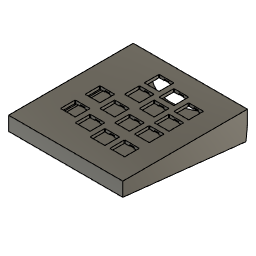
fdmyouA (Autodesk Fusion 360 design; units mm, degrees)
Autodesk Fusion 360 part; units mm, degrees
(part 1 of 2)
sketch "スケッチ1" plane through (0, 0, 0) normal (0, 0, 1) x (1, 0, 0)
  arc A0 (50.4, -11.9) -> (49.9, -12.4) centre (50.4, -12.4) ccw
  arc A1 (64.1, -12.4) -> (63.6, -11.9) centre (63.6, -12.4) ccw
  line L0 (31.4, -7.15) -> (44.6, -7.15)
  line L1 (45.1, -7.65) -> (45.1, -20.85)
  line L2 (50.4, -11.9) -> (63.6, -11.9)
  line L3 (31.4, -21.35) -> (44.6, -21.35)
  line L4 (64.1, -12.4) -> (64.1, -25.6)
  arc A2 (44.6, -21.35) -> (45.1, -20.85) centre (44.6, -20.85) ccw
  arc A3 (31.4, -7.15) -> (30.9, -7.65) centre (31.4, -7.65) ccw
  arc A4 (45.1, -7.65) -> (44.6, -7.15) centre (44.6, -7.65) ccw
  line L5 (49.9, -12.4) -> (49.9, -25.6)
  arc A5 (30.9, -20.85) -> (31.4, -21.35) centre (31.4, -20.85) ccw
  arc A6 (82.6, -30.85) -> (83.1, -30.35) centre (82.6, -30.35) ccw
  line L6 (50.4, -26.1) -> (63.6, -26.1)
  line L7 (83.1, -17.15) -> (83.1, -30.35)
  line L8 (30.9, -26.65) -> (30.9, -39.85)
  line L9 (45.1, -26.65) -> (45.1, -39.85)
  line L10 (50.4, -30.9) -> (63.6, -30.9)
  line L11 (30.9, -7.65) -> (30.9, -20.85)
  arc A7 (64.1, -31.4) -> (63.6, -30.9) centre (63.6, -31.4) ccw
  line L12 (69.4, -35.65) -> (82.6, -35.65)
  arc A8 (45.1, -26.65) -> (44.6, -26.15) centre (44.6, -26.65) ccw
  arc A9 (68.9, -30.35) -> (69.4, -30.85) centre (69.4, -30.35) ccw
  line L13 (68.9, -17.15) -> (68.9, -30.35)
  arc A10 (63.6, -26.1) -> (64.1, -25.6) centre (63.6, -25.6) ccw
  line L14 (49.9, -31.4) -> (49.9, -44.6)
  arc A11 (83.1, -17.15) -> (82.6, -16.65) centre (82.6, -17.15) ccw
  arc A12 (30.9, -39.85) -> (31.4, -40.35) centre (31.4, -39.85) ccw
  line L15 (69.4, -16.65) -> (82.6, -16.65)
  line L16 (69.4, -49.85) -> (82.6, -49.85)
  line L17 (69.4, -30.85) -> (82.6, -30.85)
  line L18 (68.9, -36.15) -> (68.9, -49.35)
  arc A13 (69.4, -35.65) -> (68.9, -36.15) centre (69.4, -36.15) ccw
  line L19 (64.1, -31.4) -> (64.1, -44.6)
  line L20 (83.1, -36.15) -> (83.1, -49.35)
  arc A14 (83.1, -36.15) -> (82.6, -35.65) centre (82.6, -36.15) ccw
  arc A15 (68.9, -49.35) -> (69.4, -49.85) centre (69.4, -49.35) ccw
  arc A16 (50.4, -30.9) -> (49.9, -31.4) centre (50.4, -31.4) ccw
  arc A17 (63.6, -45.1) -> (64.1, -44.6) centre (63.6, -44.6) ccw
  arc A18 (82.6, -49.85) -> (83.1, -49.35) centre (82.6, -49.35) ccw
  line L21 (12.4, -45.15) -> (25.6, -45.15)
  arc A19 (69.4, -16.65) -> (68.9, -17.15) centre (69.4, -17.15) ccw
  arc A20 (44.6, -40.35) -> (45.1, -39.85) centre (44.6, -39.85) ccw
  line L22 (31.4, -26.15) -> (44.6, -26.15)
  arc A21 (31.4, -26.15) -> (30.9, -26.65) centre (31.4, -26.65) ccw
  arc A22 (49.9, -25.6) -> (50.4, -26.1) centre (50.4, -25.6) ccw
  arc A23 (49.9, -44.6) -> (50.4, -45.1) centre (50.4, -44.6) ccw
  line L23 (31.4, -40.35) -> (44.6, -40.35)
  line L24 (50.4, -92.6) -> (63.6, -92.6)
  line L25 (49.9, -55.15) -> (49.9, -68.35)
  line L26 (69.4, -54.65) -> (82.6, -54.65)
  arc A24 (82.6, -92.6) -> (83.1, -92.1) centre (82.6, -92.1) ccw
  line L27 (83.1, -55.15) -> (83.1, -68.35)
  arc A25 (26.1, -69.4) -> (25.6, -68.9) centre (25.6, -69.4) ccw
  arc A26 (44.6, -87.85) -> (45.1, -87.35) centre (44.6, -87.35) ccw
  line L28 (64.1, -55.15) -> (64.1, -68.35)
  arc A27 (31.4, -49.9) -> (30.9, -50.4) centre (31.4, -50.4) ccw
  arc A28 (11.9, -58.85) -> (12.4, -59.35) centre (12.4, -58.85) ccw
  line L29 (31.4, -64.1) -> (44.6, -64.1)
  line L30 (69.4, -68.85) -> (82.6, -68.85)
  arc A29 (30.9, -63.6) -> (31.4, -64.1) centre (31.4, -63.6) ccw
  line L31 (11.9, -45.65) -> (11.9, -58.85)
  line L32 (12.4, -68.9) -> (25.6, -68.9)
  arc A30 (12.4, -45.15) -> (11.9, -45.65) centre (12.4, -45.65) ccw
  line L33 (31.4, -49.9) -> (44.6, -49.9)
  line L34 (12.4, -83.1) -> (25.6, -83.1)
  arc A31 (26.1, -45.65) -> (25.6, -45.15) centre (25.6, -45.65) ccw
  line L35 (68.9, -55.15) -> (68.9, -68.35)
  arc A32 (11.9, -82.6) -> (12.4, -83.1) centre (12.4, -82.6) ccw
  arc A33 (45.1, -50.4) -> (44.6, -49.9) centre (44.6, -50.4) ccw
  arc A34 (44.6, -64.1) -> (45.1, -63.6) centre (44.6, -63.6) ccw
  line L36 (12.4, -59.35) -> (25.6, -59.35)
  arc A35 (82.6, -68.85) -> (83.1, -68.35) centre (82.6, -68.35) ccw
  arc A36 (68.9, -68.35) -> (69.4, -68.85) centre (69.4, -68.35) ccw
  arc A37 (49.9, -68.35) -> (50.4, -68.85) centre (50.4, -68.35) ccw
  line L37 (50.4, -54.65) -> (63.6, -54.65)
  arc A38 (63.6, -68.85) -> (64.1, -68.35) centre (63.6, -68.35) ccw
  line L38 (30.9, -74.15) -> (30.9, -87.35)
  arc A39 (31.4, -73.65) -> (30.9, -74.15) centre (31.4, -74.15) ccw
  arc A40 (64.1, -55.15) -> (63.6, -54.65) centre (63.6, -55.15) ccw
  line L39 (31.4, -87.85) -> (44.6, -87.85)
  arc A41 (50.4, -54.65) -> (49.9, -55.15) centre (50.4, -55.15) ccw
  line L40 (26.1, -45.65) -> (26.1, -58.85)
  line L41 (45.1, -74.15) -> (45.1, -87.35)
  line L42 (45.1, -50.4) -> (45.1, -63.6)
  line L43 (50.4, -68.85) -> (63.6, -68.85)
  line L44 (50.4, -78.4) -> (63.6, -78.4)
  arc A42 (69.4, -54.65) -> (68.9, -55.15) centre (69.4, -55.15) ccw
  arc A43 (45.1, -74.15) -> (44.6, -73.65) centre (44.6, -74.15) ccw
  line L45 (64.1, -78.9) -> (64.1, -92.1)
  arc A44 (50.4, -78.4) -> (49.9, -78.9) centre (50.4, -78.9) ccw
  arc A45 (12.4, -68.9) -> (11.9, -69.4) centre (12.4, -69.4) ccw
  arc A46 (25.6, -83.1) -> (26.1, -82.6) centre (25.6, -82.6) ccw
  arc A47 (25.6, -59.35) -> (26.1, -58.85) centre (25.6, -58.85) ccw
  line L46 (30.9, -50.4) -> (30.9, -63.6)
  arc A48 (83.1, -55.15) -> (82.6, -54.65) centre (82.6, -55.15) ccw
  line L47 (11.9, -69.4) -> (11.9, -82.6)
  line L48 (26.1, -69.4) -> (26.1, -82.6)
  line L49 (31.4, -73.65) -> (44.6, -73.65)
  line L50 (49.9, -78.9) -> (49.9, -92.1)
  arc A49 (64.1, -78.9) -> (63.6, -78.4) centre (63.6, -78.9) ccw
  arc A50 (30.9, -87.35) -> (31.4, -87.85) centre (31.4, -87.35) ccw
  line L51 (69.4, -92.6) -> (82.6, -92.6)
  arc A51 (63.6, -92.6) -> (64.1, -92.1) centre (63.6, -92.1) ccw
  line L52 (69.4, -78.4) -> (82.6, -78.4)
  line L53 (83.1, -78.9) -> (83.1, -92.1)
  arc A52 (69.4, -78.4) -> (68.9, -78.9) centre (69.4, -78.9) ccw
  arc A53 (49.9, -92.1) -> (50.4, -92.6) centre (50.4, -92.1) ccw
  arc A54 (68.9, -92.1) -> (69.4, -92.6) centre (69.4, -92.1) ccw
  line L54 (68.9, -78.9) -> (68.9, -92.1)
  arc A55 (83.1, -78.9) -> (82.6, -78.4) centre (82.6, -78.9) ccw
  line L55 (-2.5, -3.7) -> (97.5, -3.7)
  line L56 (-7.5, -3.7) -> (102.5, -3.7)
  line L57 (102.5, -3.7) -> (102.5, -113.7)
  line L58 (102.5, -113.7) -> (-7.5, -113.7)
  line L59 (-7.5, -113.7) -> (-7.5, -3.7)
  line L60 (47.5, -3.7) -> (47.5, -113.7)
  line L61 (47.5, -3.7) -> (42.3, -3.7)
  line L62 (47.5, -3.7) -> (-2.7, -3.7)
  line L63 (-2.7, -3.7) -> (97.7, -3.7)
  line L64 (97.7, -3.7) -> (97.7, -103.9)
  line L65 (97.7, -103.9) -> (-2.7, -103.9)
  line L66 (-2.7, -103.9) -> (-2.7, -3.7)
  line L67 (47.5, -3.7) -> (9.5, -3.7)
  line L68 (9.5, -3.7) -> (7.4071, -3.7)
  line L69 (-2.7, -3.7) -> (7.3, -3.7)
  line L70 (7.3, -3.7) -> (7.3, -103.9)
  line L71 (7.3, -103.9) -> (-2.7, -103.9)
  line L72 (-2.7, -103.9) -> (-2.7, 6.3)
  line L73 (-2.7, -103.9) -> (97.7, -103.9)
  line L74 (97.7, -103.9) -> (97.7, -93.9)
  line L75 (97.7, -93.9) -> (-2.7, -93.9)
  line L76 (-2.7, -93.9) -> (-2.7, -103.9)
  line L77 (97.7, -103.9) -> (87.7, -103.9)
  line L78 (87.7, -103.9) -> (87.7, -3.7)
  line L79 (87.7, -3.7) -> (97.7, -3.7)
  line L80 (97.7, -3.7) -> (97.7, -103.9)
  line L81 (40.1, -21.85) -> (35.9, -21.85)
  line L82 (35.9, -21.85) -> (35.9, -21.35)
  line L83 (40.1, -21.35) -> (40.1, -21.85)
  line L84 (40.1, -21.85) -> (38, -21.35) construction
  line L85 (35.9, -21.85) -> (38, -21.35) construction
  line L86 (38, -7.15) -> (40.1, -6.65) construction
  line L87 (38, -7.15) -> (35.9, -6.65) construction
  line L88 (40.1, -6.65) -> (40.1, -7.15)
  line L89 (35.9, -7.65) -> (35.9, -6.65)
  line L90 (35.9, -6.65) -> (40.1, -6.65)
  line L91 (35.9, -7.15) -> (35.9, -6.65)
  line L92 (38, -7.15) -> (40.1, -6.65) construction
  line L93 (35.9, -6.65) -> (40.1, -6.65)
  line L94 (38, -7.15) -> (35.9, -6.65) construction
  line L95 (40.1, -6.65) -> (40.1, -7.15)
  line L96 (54.9, -11.9) -> (54.9, -11.4)
  line L97 (57, -11.9) -> (59.1, -11.4) construction
  line L98 (54.9, -11.4) -> (59.1, -11.4)
  line L99 (57, -11.9) -> (54.9, -11.4) construction
  line L100 (59.1, -11.4) -> (59.1, -12.4)
  line L101 (54.9, -26.6) -> (54.9, -26.1)
  line L102 (54.9, -26.6) -> (57, -26.1) construction
  line L103 (59.1, -26.6) -> (54.9, -26.6)
  line L104 (59.1, -26.1) -> (59.1, -26.6)
  line L105 (73.9, -16.65) -> (73.9, -16.15)
  line L106 (76, -16.65) -> (78.1, -16.15) construction
  line L107 (73.9, -16.15) -> (78.1, -16.15)
  line L108 (76, -16.65) -> (73.9, -16.15) construction
  line L109 (78.1, -16.15) -> (78.1, -16.65)
  line L110 (73.9, -31.35) -> (73.9, -30.85)
  line L111 (73.9, -31.35) -> (76, -30.85) construction
  line L112 (78.1, -31.35) -> (73.9, -31.35)
  line L113 (78.1, -31.35) -> (76, -30.85) construction
  line L114 (78.1, -30.85) -> (78.1, -31.35)
  line L115 (35.9, -26.15) -> (35.9, -25.65)
  line L116 (38, -26.15) -> (40.1, -25.65) construction
  line L117 (35.9, -25.65) -> (40.1, -25.65)
  line L118 (38, -26.15) -> (35.9, -25.65) construction
  line L119 (40.1, -25.65) -> (40.1, -26.15)
  line L120 (35.9, -40.85) -> (35.9, -40.35)
  line L121 (40.1, -40.85) -> (35.9, -40.85)
  line L122 (40.1, -40.85) -> (38, -40.35) construction
  line L123 (40.1, -40.35) -> (40.1, -40.85)
  line L124 (54.9, -30.9) -> (54.9, -30.4)
  line L125 (57, -30.9) -> (59.1, -30.4) construction
  line L126 (54.9, -30.4) -> (59.1, -30.4)
  line L127 (57, -30.9) -> (54.9, -30.4) construction
  line L128 (59.1, -30.4) -> (59.1, -30.9)
  line L129 (54.9, -45.6) -> (54.9, -45.1)
  line L130 (54.9, -45.6) -> (57, -45.1) construction
  line L131 (59.1, -45.6) -> (54.9, -45.6)
  line L132 (59.1, -45.6) -> (57, -45.1) construction
  line L133 (59.1, -45.1) -> (59.1, -45.6)
  line L134 (73.9, -35.65) -> (73.9, -35.15)
  line L135 (76, -35.65) -> (78.1, -35.15) construction
  line L136 (73.9, -35.15) -> (78.1, -35.15)
  line L137 (76, -35.65) -> (73.9, -35.15) construction
  line L138 (78.1, -35.15) -> (78.1, -35.65)
  line L139 (73.9, -50.35) -> (73.9, -49.85)
  line L140 (73.9, -50.35) -> (76, -49.85) construction
  line L141 (78.1, -50.35) -> (73.9, -50.35)
  line L142 (78.1, -50.35) -> (76, -49.85) construction
  line L143 (78.1, -49.85) -> (78.1, -50.35)
  line L144 (16.9, -45.15) -> (16.9, -44.65)
  line L145 (16.9, -45.65) -> (21.1, -44.65) construction
  line L146 (16.9, -44.65) -> (21.1, -44.65)
  line L147 (19, -45.15) -> (16.9, -44.65) construction
  line L148 (21.1, -44.65) -> (21.1, -45.15)
  line L149 (16.9, -59.85) -> (16.9, -59.35)
  line L150 (16.9, -59.85) -> (19, -59.35) construction
  line L151 (21.1, -59.85) -> (16.9, -59.85)
  line L152 (21.1, -59.85) -> (19, -59.35) construction
  line L153 (21.1, -59.35) -> (21.1, -59.85)
  line L154 (35.9, -49.9) -> (35.9, -49.4)
  line L155 (38, -49.9) -> (40.1, -49.4) construction
  line L156 (35.9, -49.4) -> (40.1, -49.4)
  line L157 (38, -49.9) -> (35.9, -49.4) construction
  line L158 (40.1, -49.4) -> (40.1, -49.9)
  line L159 (35.9, -64.6) -> (35.9, -64.1)
  line L160 (35.9, -64.6) -> (38, -64.1) construction
  line L161 (40.1, -64.6) -> (35.9, -64.6)
  line L162 (40.1, -64.6) -> (38, -64.1) construction
  line L163 (40.1, -64.1) -> (40.1, -64.6)
  line L164 (54.9, -54.65) -> (54.9, -54.15)
  line L165 (57, -54.65) -> (59.1, -54.15) construction
  line L166 (54.9, -54.15) -> (59.1, -54.15)
  line L167 (57, -54.65) -> (54.9, -54.15) construction
  line L168 (59.1, -54.15) -> (59.1, -54.65)
  line L169 (54.9, -69.35) -> (54.9, -68.85)
  line L170 (54.9, -69.35) -> (57, -68.85) construction
  line L171 (59.1, -69.35) -> (54.9, -69.35)
  line L172 (59.1, -69.35) -> (57, -68.85) construction
  line L173 (59.1, -68.85) -> (59.1, -69.35)
  line L174 (73.9, -54.65) -> (73.9, -54.15)
  line L175 (73.9, -54.15) -> (78.1, -54.15)
  line L176 (78.1, -55.15) -> (73.9, -54.15) construction
  line L177 (78.1, -54.15) -> (78.1, -54.65)
  line L178 (73.9, -69.35) -> (73.9, -68.85)
  line L179 (73.9, -69.35) -> (76, -68.85) construction
  line L180 (78.1, -69.35) -> (73.9, -69.35)
  line L181 (78.1, -69.35) -> (76, -68.85) construction
  line L182 (78.1, -68.85) -> (78.1, -69.35)
  line L183 (16.9, -68.9) -> (16.9, -68.4)
  line L184 (19, -68.9) -> (21.1, -68.4) construction
  line L185 (16.9, -68.4) -> (21.1, -68.4)
  line L186 (19, -68.9) -> (16.9, -68.4) construction
  line L187 (21.1, -68.4) -> (21.1, -68.9)
  line L188 (16.9, -83.6) -> (16.9, -83.1)
  line L189 (16.9, -83.6) -> (19, -83.1) construction
  line L190 (21.1, -83.6) -> (16.9, -83.6)
  line L191 (21.1, -83.6) -> (19, -83.1) construction
  line L192 (21.1, -83.1) -> (21.1, -83.6)
  line L193 (35.9, -88.35) -> (35.9, -87.85)
  line L194 (35.9, -88.35) -> (38, -87.85) construction
  line L195 (40.1, -88.35) -> (35.9, -88.35)
  line L196 (40.1, -88.35) -> (38, -87.85) construction
  line L197 (40.1, -87.85) -> (40.1, -88.35)
  line L198 (54.9, -78.4) -> (54.9, -77.9)
  line L199 (57, -78.4) -> (59.1, -77.9) construction
  line L200 (54.9, -77.9) -> (59.1, -77.9)
  line L201 (57, -78.4) -> (54.9, -77.9) construction
  line L202 (59.1, -77.9) -> (59.1, -78.4)
  line L203 (54.9, -93.1) -> (54.9, -92.6)
  line L204 (54.9, -93.1) -> (57, -92.6) construction
  line L205 (59.1, -93.1) -> (54.9, -93.1)
  line L206 (59.1, -93.1) -> (57, -92.6) construction
  line L207 (59.1, -92.6) -> (59.1, -93.1)
  line L208 (73.9, -78.4) -> (73.9, -77.9)
  line L209 (76, -78.4) -> (78.1, -77.9) construction
  line L210 (73.9, -77.9) -> (78.1, -77.9)
  line L211 (76, -78.4) -> (73.9, -77.9) construction
  line L212 (78.1, -77.9) -> (78.1, -78.4)
  line L213 (73.9, -93.1) -> (73.9, -92.6)
  line L214 (78.1, -93.1) -> (73.9, -93.1)
  line L215 (78.1, -93.1) -> (76, -92.6) construction
  line L216 (78.1, -92.6) -> (78.1, -93.1)
  line L217 (35.9, -88.35) -> (35.9, -87.85)
  line L218 (40.1, -87.85) -> (40.1, -88.35)
  line L219 (40.1, -88.35) -> (38, -87.85) construction
  line L220 (40.1, -88.35) -> (35.9, -88.35)
  line L221 (35.9, -88.35) -> (38, -87.85) construction
  line L222 (35.9, -73.65) -> (35.9, -73.15)
  line L223 (35.9, -73.15) -> (40.1, -73.15)
  line L224 (40.1, -73.15) -> (40.1, -73.65)
  line L225 (38, -73.65) -> (35.9, -73.15) construction
  line L226 (38, -73.65) -> (40.1, -73.15) construction
  line L227 (76, -54.65) -> (76, -55.15)
  line L228 (49.9, -45.1) -> (63.6, -45.1)
  line L229 (38, -7.15) -> (38, -21.35)
  line L230 (45.1, -14.25) -> (30.9, -14.25)
  line L231 (57, -11.9) -> (57, -26.1)
  line L232 (49.9, -19) -> (64.1, -19)
  line L233 (76, -16.65) -> (76, -30.85)
  line L234 (68.9, -23.75) -> (83.1, -23.75)
  line L235 (76, -35.65) -> (76, -49.85)
  line L236 (83.1, -42.75) -> (68.9, -42.75)
  line L237 (76, -54.65) -> (76, -68.85)
  line L238 (83.1, -61.75) -> (68.9, -61.75)
  line L239 (76, -78.4) -> (76, -92.6)
  line L240 (83.1, -85.5) -> (68.9, -85.5)
  line L241 (64.1, -85.5) -> (49.9, -85.5)
  line L242 (57, -78.4) -> (57, -92.6)
  line L243 (57, -68.85) -> (57, -54.65)
  line L244 (64.1, -61.75) -> (49.9, -61.75)
  line L245 (64.1, -38) -> (49.9, -38)
  line L246 (57, -30.9) -> (57, -45.1)
  line L247 (45.1, -33.25) -> (30.9, -33.25)
  line L248 (38, -26.15) -> (38, -40.35)
  line L249 (45.1, -57) -> (30.9, -57)
  line L250 (38, -49.9) -> (38, -64.1)
  line L251 (38, -73.65) -> (38, -87.85)
  line L252 (45.1, -80.75) -> (30.9, -80.75)
  line L253 (19, -68.9) -> (19, -83.1)
  line L254 (26.1, -76) -> (11.9, -76)
  line L255 (76, -85.5) -> (76, -92.6)
  line L256 (38, -80.75) -> (38, -87.85)
  line L257 (19, -76) -> (19, -83.1)
  line L258 (47.5, -23.75) -> (28.5, -23.75)
  line L259 (28.5, -23.75) -> (28.5, -4.75)
  line L260 (28.5, -4.75) -> (47.5, -4.75)
  line L261 (47.5, -4.75) -> (47.5, -23.75)
  line L262 (47.5, -23.75) -> (28.5, -4.75) construction
  line L263 (28.5, -23.75) -> (47.5, -4.75) construction
  line L264 (66.5, -28.5) -> (47.5, -28.5)
  line L265 (47.5, -28.5) -> (47.5, -9.5)
  line L266 (47.5, -9.5) -> (66.5, -9.5)
  line L267 (66.5, -9.5) -> (66.5, -28.5)
  line L268 (66.5, -28.5) -> (47.5, -9.5) construction
  line L269 (47.5, -28.5) -> (66.5, -9.5) construction
  line L270 (85.5, -33.25) -> (66.5, -33.25)
  line L271 (66.5, -33.25) -> (66.5, -14.25)
  line L272 (66.5, -14.25) -> (85.5, -14.25)
  line L273 (85.5, -14.25) -> (85.5, -33.25)
  line L274 (85.5, -33.25) -> (66.5, -14.25) construction
  line L275 (66.5, -33.25) -> (85.5, -14.25) construction
  line L276 (85.5, -33.25) -> (66.5, -33.25)
  line L277 (66.5, -33.25) -> (66.5, -52.25)
  line L278 (66.5, -52.25) -> (85.5, -52.25)
  line L279 (85.5, -52.25) -> (85.5, -33.25)
  line L280 (85.5, -33.25) -> (66.5, -52.25) construction
  line L281 (66.5, -33.25) -> (85.5, -52.25) construction
  line L282 (47.5, -47.5) -> (66.5, -47.5)
  line L283 (66.5, -47.5) -> (66.5, -28.5)
  line L284 (66.5, -28.5) -> (47.5, -28.5)
  line L285 (47.5, -28.5) -> (47.5, -47.5)
  line L286 (47.5, -47.5) -> (66.5, -28.5) construction
  line L287 (66.5, -47.5) -> (47.5, -28.5) construction
  line L288 (47.5, -42.75) -> (28.5, -42.75)
  line L289 (28.5, -42.75) -> (28.5, -23.75)
  line L290 (28.5, -23.75) -> (47.5, -23.75)
  line L291 (47.5, -23.75) -> (47.5, -42.75)
  line L292 (47.5, -42.75) -> (28.5, -23.75) construction
  line L293 (28.5, -42.75) -> (47.5, -23.75) construction
  line L294 (47.5, -66.5) -> (28.5, -66.5)
  line L295 (28.5, -66.5) -> (28.5, -47.5)
  line L296 (28.5, -47.5) -> (47.5, -47.5)
  line L297 (47.5, -47.5) -> (47.5, -66.5)
  line L298 (47.5, -66.5) -> (28.5, -47.5) construction
  line L299 (28.5, -66.5) -> (47.5, -47.5) construction
  line L300 (11.9, -52.25) -> (26.1, -52.25)
  line L301 (19, -45.15) -> (19, -59.35)
  line L302 (28.5, -61.75) -> (9.5, -61.75)
  line L303 (9.5, -61.75) -> (9.5, -42.75)
  line L304 (9.5, -42.75) -> (28.5, -42.75)
  line L305 (28.5, -42.75) -> (28.5, -61.75)
  line L306 (28.5, -61.75) -> (9.5, -42.75) construction
  line L307 (9.5, -61.75) -> (28.5, -42.75) construction
  line L308 (28.5, -85.5) -> (9.5, -85.5)
  line L309 (9.5, -85.5) -> (9.5, -66.5)
  line L310 (9.5, -66.5) -> (28.5, -66.5)
  line L311 (28.5, -66.5) -> (28.5, -85.5)
  line L312 (28.5, -85.5) -> (9.5, -66.5) construction
  line L313 (9.5, -85.5) -> (28.5, -66.5) construction
  line L314 (47.5, -90.7675) -> (28.5, -90.7675)
  line L315 (28.5, -90.7675) -> (28.5, -71.7675)
  line L316 (28.5, -71.7675) -> (47.5, -71.7675)
  line L317 (47.5, -71.7675) -> (47.5, -90.7675)
  line L318 (47.5, -90.7675) -> (28.5, -71.7675) construction
  line L319 (28.5, -90.7675) -> (47.5, -71.7675) construction
  line L320 (66.5, -95) -> (47.5, -95)
  line L321 (47.5, -95) -> (47.5, -76)
  line L322 (47.5, -76) -> (66.5, -76)
  line L323 (66.5, -76) -> (66.5, -95)
  line L324 (66.5, -95) -> (47.5, -76) construction
  line L325 (47.5, -95) -> (66.5, -76) construction
  line L326 (85.5, -95) -> (66.5, -95)
  line L327 (66.5, -95) -> (66.5, -76)
  line L328 (66.5, -76) -> (85.5, -76)
  line L329 (85.5, -76) -> (85.5, -95)
  line L330 (85.5, -95) -> (66.5, -76) construction
  line L331 (66.5, -95) -> (85.5, -76) construction
  line L332 (66.5, -71.25) -> (47.5, -71.25)
  line L333 (47.5, -71.25) -> (47.5, -52.25)
  line L334 (47.5, -52.25) -> (66.5, -52.25)
  line L335 (66.5, -52.25) -> (66.5, -71.25)
  line L336 (66.5, -71.25) -> (47.5, -52.25) construction
  line L337 (47.5, -71.25) -> (66.5, -52.25) construction
  line L338 (85.5, -71.25) -> (66.5, -71.25)
  line L339 (66.5, -71.25) -> (66.5, -52.25)
  line L340 (66.5, -52.25) -> (85.5, -52.25)
  line L341 (85.5, -52.25) -> (85.5, -71.25)
  line L342 (85.5, -71.25) -> (66.5, -52.25) construction
  line L343 (66.5, -71.25) -> (85.5, -52.25) construction
  line L344 (-7.5, -3.7) -> (102.5, -3.7)
  line L345 (102.5, -3.7) -> (102.5, 6.3)
  line L346 (102.5, 6.3) -> (-7.5, 6.3)
  line L347 (-7.5, 6.3) -> (-7.5, -3.7)
  line L348 (7.3, -3.7) -> (7.3, 6.3)
  line L349 (87.7, -3.7) -> (87.7, 6.3)
  line L350 (97.7, -3.7) -> (97.7, 6.3)
  line L351 (26.5, -23.75) -> (26.5, -3.7)
  line L352 (-2.7, -40.75) -> (26.5, -40.75)
  line L353 (26.5, -23.75) -> (26.5, -40.75)
  point P0 (38, -21.35)
  point P1 (38, -7.15)
  point P2 (38, -7.15)
  point P3 (38, -7.15)
  point P4 (38, -7.15)
  point P5 (38, -7.15)
  point P6 (57, -11.9)
  point P7 (57, -11.9)
  point P8 (57, -26.1)
  point P9 (57, -26.1)
  point P10 (76, -16.65)
  point P11 (76, -16.65)
  point P12 (76, -30.85)
  point P13 (76, -30.85)
  point P14 (38, -26.15)
  point P15 (38, -26.15)
  point P16 (38, -40.35)
  point P17 (38, -40.35)
  point P18 (57, -30.9)
  point P19 (57, -45.1)
  point P20 (57, -45.1)
  point P21 (76, -35.65)
  point P22 (76, -35.65)
  point P23 (76, -49.85)
  point P24 (76, -49.85)
  point P25 (19, -45.15)
  point P26 (19, -45.15)
  point P27 (19, -59.35)
  point P28 (19, -59.35)
  point P29 (38, -49.9)
  point P30 (38, -49.9)
  point P31 (38, -64.1)
  point P32 (38, -64.1)
  point P33 (57, -54.65)
  point P34 (57, -54.65)
  point P35 (57, -68.85)
  point P36 (57, -68.85)
  point P37 (76, -54.65)
  point P38 (76, -54.65)
  point P39 (76, -68.85)
  point P40 (76, -68.85)
  point P41 (19, -68.9)
  point P42 (19, -68.9)
  point P43 (19, -83.1)
  point P44 (19, -83.1)
  point P45 (38, -87.85)
  point P46 (38, -87.85)
  point P47 (57, -78.4)
  point P48 (57, -78.4)
  point P49 (57, -92.6)
  point P50 (57, -92.6)
  point P51 (76, -78.4)
  point P52 (76, -78.4)
  point P53 (76, -92.6)
  point P54 (76, -92.6)
  point P55 (38, -87.85)
  point P56 (38, -87.85)
  point P57 (38, -87.85)
  point P58 (38, -87.85)
  point P59 (38, -73.65)
  point P60 (38, -73.65)
  point P61 (38, -73.65)
  point P62 (38, -73.65)
  point P63 (38, -14.25)
  point P64 (57, -19)
  point P65 (76, -23.75)
  point P66 (76, -42.75)
  point P67 (57, -38)
  point P68 (38, -33.25)
  point P69 (38, -57)
  point P70 (19, -52.25)
  point P71 (19, -76)
  point P72 (38, -81.2675)
  point P73 (57, -85.5)
  point P74 (76, -85.5)
  point P75 (57, -61.75)
  point P76 (76, -61.75)
  dimension "d8" = 110
  dimension "d9" = 110
  dimension "d11" = 50.2
  dimension "d12" = 100.4
  dimension "d13" = 100.2
  dimension "d15" = 10
  dimension "d16" = 100.4
  dimension "d17" = 10
  dimension "d18" = 10
  dimension "d19" = 100.2
  dimension "d22" = 4.2
  dimension "d23" = 1
  dimension "d24" = 4.2
  dimension "d26" = 4.2
  dimension "d30" = 4.2
  dimension "d34" = 4.2
  dimension "d38" = 4.2
  dimension "d42" = 4.2
  dimension "d46" = 4.2
  dimension "d47" = 1
  dimension "d50" = 4.2
  dimension "d54" = 4.2
  dimension "d58" = 4.2
  dimension "d62" = 4.2
  dimension "d68" = 4.2
  dimension "d72" = 4.2
  dimension "d78" = 4.2
  dimension "d97" = 19
  dimension "d98" = 19
  dimension "d99" = 19
  dimension "d100" = 19
  dimension "d101" = 19
  dimension "d102" = 19
  dimension "d103" = 19
  dimension "d104" = 19
  dimension "d105" = 19
  dimension "d106" = 19
  dimension "d107" = 19
  dimension "d108" = 19
  dimension "d109" = 19
  dimension "d110" = 19
  dimension "d111" = 19
  dimension "d112" = 19
  dimension "d113" = 19
  dimension "d114" = 19
  dimension "d115" = 19
  dimension "d116" = 19
  dimension "d117" = 19
  dimension "d118" = 19
  dimension "d119" = 19
  dimension "d120" = 19
  dimension "d121" = 19
  dimension "d122" = 19
  dimension "d123" = 19
  dimension "d124" = 19
  dimension "d127" = 110
  dimension "d128" = 10
  dimension "d144" = 8.9
  dimension "d145" = 9.8
  dimension "d152" = 12.2
  dimension "d153" = 4.8
  constraint midpoint L55 L56
  constraint vertical L57
  constraint horizontal L58
  constraint vertical L59
  constraint midpoint L56 L60.start
  constraint perpendicular L58 L60
  constraint coincident L58 L60.end
  constraint perpendicular L60 L61
  constraint perpendicular L60 L62
  constraint horizontal L63
  constraint vertical L64
  constraint horizontal L65
  constraint vertical L66
  constraint perpendicular L60 L67
  constraint coincident L62 L68.end
  constraint coincident L56 L68.end
  constraint horizontal L69
  constraint vertical L70
  constraint horizontal L71
  constraint vertical L72
  constraint coincident L65 L70.end
  constraint horizontal L73
  constraint vertical L74
  constraint horizontal L75
  constraint vertical L76
  constraint horizontal L77
  constraint vertical L78
  constraint horizontal L79
  constraint vertical L80
  constraint midpoint L0 P5
  constraint midpoint L3 P0
  constraint horizontal L81
  constraint perpendicular L81 L82
  constraint parallel L82 L83
  constraint coincident L84 P0
  constraint coincident L85 P0
  constraint coincident P0 L84.end
  constraint parallel L88 L89
  constraint coincident P5 L87
  constraint coincident P5 L86
  constraint coincident P5 P4
  constraint parallel L91 L95
  constraint coincident P5 L94
  constraint coincident P5 L92
  constraint parallel L96 L100
  constraint coincident P7 L99
  constraint coincident P7 L97
  constraint coincident P7 P6
  constraint horizontal L103
  constraint perpendicular L101 L103
  constraint parallel L101 L104
  constraint coincident P9 L102
  constraint coincident P9 P8
  constraint parallel L105 L109
  constraint coincident P11 L108
  constraint coincident P11 L106
  constraint coincident P11 P10
  constraint horizontal L112
  constraint perpendicular L110 L112
  constraint parallel L110 L114
  constraint coincident P13 L113
  constraint coincident P13 L111
  constraint coincident P13 P12
  constraint parallel L115 L119
  constraint coincident P15 L118
  constraint coincident P15 L116
  constraint coincident P15 P14
  constraint horizontal L121
  constraint perpendicular L120 L121
  constraint parallel L120 L123
  constraint coincident P17 L122
  constraint coincident P17 P16
  constraint parallel L124 L128
  constraint coincident P18 L125.start
  constraint horizontal L131
  constraint perpendicular L129 L131
  constraint parallel L129 L133
  constraint coincident P20 L132
  constraint coincident P20 L130
  constraint coincident P20 P19
  constraint parallel L134 L138
  constraint coincident P22 L137
  constraint coincident P22 L135
  constraint coincident P22 P21
  constraint horizontal L141
  constraint perpendicular L139 L141
  constraint parallel L139 L143
  constraint coincident P24 L142
  constraint coincident P24 L140
  constraint coincident P24 P23
  constraint parallel L144 L148
  constraint coincident P26 L147
  constraint coincident P26 L145
  constraint coincident P26 P25
  constraint horizontal L151
  constraint perpendicular L149 L151
  constraint parallel L149 L153
  constraint coincident P28 L152
  constraint coincident P28 L150
  constraint coincident P28 P27
  constraint parallel L154 L158
  constraint coincident P30 L157
  constraint coincident P30 L155
  constraint coincident P30 P29
  constraint horizontal L161
  constraint perpendicular L159 L161
  constraint parallel L159 L163
  constraint coincident P32 L162
  constraint coincident P32 L160
  constraint coincident P32 P31
  constraint parallel L164 L168
  constraint coincident P34 L167
  constraint coincident P34 L165
  constraint coincident P34 P33
  constraint horizontal L171
  constraint perpendicular L169 L171
  constraint parallel L169 L173
  constraint coincident P36 L172
  constraint coincident P36 L170
  constraint coincident P36 P35
  constraint parallel L174 L177
  constraint coincident P38 L176
  constraint coincident P38 P37
  constraint horizontal L180
  constraint perpendicular L178 L180
  constraint parallel L178 L182
  constraint coincident P40 L181
  constraint coincident P40 L179
  constraint coincident P40 P39
  constraint parallel L183 L187
  constraint coincident P42 L186
  constraint coincident P42 L184
  constraint coincident P42 P41
  constraint horizontal L190
  constraint perpendicular L188 L190
  constraint parallel L188 L192
  constraint coincident P44 L191
  constraint coincident P44 L189
  constraint coincident P44 P43
  constraint horizontal L195
  constraint perpendicular L193 L195
  constraint parallel L193 L197
  constraint coincident P58 L196
  constraint coincident P58 L194
  constraint coincident P58 P57
  constraint parallel L198 L202
  constraint coincident P48 L201
  constraint coincident P48 L199
  constraint coincident P48 P47
  constraint horizontal L205
  constraint perpendicular L203 L205
  constraint parallel L203 L207
  constraint coincident P50 L206
  constraint coincident P50 L204
  constraint coincident P50 P49
  constraint parallel L208 L212
  constraint coincident P52 L211
  constraint coincident P52 L209
  constraint coincident P52 P51
  constraint horizontal L214
  constraint perpendicular L213 L214
  constraint parallel L213 L216
  constraint coincident P54 L215
  constraint coincident P54 P53
  constraint midpoint L26 P38
  constraint perpendicular L30 L227
  constraint midpoint L49 P62
  constraint horizontal L220
  constraint perpendicular L217 L220
  constraint parallel L217 L218
  constraint coincident P58 L219
  constraint coincident P58 L221
  constraint parallel L222 L224
  constraint coincident P62 L225
  constraint coincident P62 L226
  constraint coincident P62 P61
  constraint coincident L15 L105.start
  constraint coincident L15 L109.end
  constraint coincident L17 L110.end
  constraint coincident L17 L114.start
  constraint coincident L12 L138.end
  constraint coincident L12 L134.start
  constraint coincident L16 L139.end
  constraint coincident L16 L143.start
  constraint coincident L26 L177.end
  constraint coincident L26 L174.start
  constraint coincident L30 L178.end
  constraint coincident L30 L182.start
  constraint coincident L52 L208.start
  constraint coincident L52 L212.end
  constraint coincident L51 L213.end
  constraint coincident L51 L216.start
  constraint coincident L24 L203.end
  constraint coincident L24 L207.start
  constraint coincident L44 L202.end
  constraint coincident L44 L198.start
  constraint coincident L43 L169.end
  constraint coincident L43 L173.start
  constraint coincident L37 L164.start
  constraint coincident L37 L168.end
  constraint coincident L228 L133.start
  constraint coincident L10 L128.end
  constraint coincident L10 L124.start
  constraint coincident L6 L101.end
  constraint coincident L6 L104.start
  constraint coincident L2 L96.start
  constraint coincident L0 L88.end
  constraint coincident L0 L91.start
  constraint coincident L3 L83.start
  constraint coincident L3 L82.end
  constraint coincident L22 L115.start
  constraint coincident L22 L119.end
  constraint coincident L23 L120.end
  constraint coincident L23 L123.start
  constraint coincident L33 L154.start
  constraint coincident L33 L158.end
  constraint coincident L29 L159.end
  constraint coincident L29 L163.start
  constraint coincident L49 L222.start
  constraint coincident L49 L224.end
  constraint coincident L39 L193.end
  constraint coincident L39 L197.start
  constraint coincident L34 L188.end
  constraint coincident L34 L192.start
  constraint coincident L32 L187.end
  constraint coincident L32 L183.start
  constraint coincident L36 L149.end
  constraint coincident L36 L153.start
  constraint coincident L21 L144.start
  constraint coincident L21 L148.end
  constraint coincident L129.end L228
  constraint coincident A23.end L228
  constraint perpendicular L3 L229
  constraint midpoint L1 L230.start
  constraint midpoint L11 L230.end
  constraint perpendicular L6 L231
  constraint midpoint L5 L232.start
  constraint midpoint L4 L232.end
  constraint perpendicular L17 L233
  constraint midpoint L13 L234.start
  constraint midpoint L7 L234.end
  constraint perpendicular L16 L235
  constraint midpoint L20 L236.start
  constraint midpoint L18 L236.end
  constraint perpendicular L30 L237
  constraint midpoint L27 L238.start
  constraint midpoint L35 L238.end
  constraint perpendicular L51 L239
  constraint midpoint L53 L240.start
  constraint midpoint L54 L240.end
  constraint midpoint L45 L241.start
  constraint midpoint L50 L241.end
  constraint perpendicular L24 L242
  constraint perpendicular L37 L243
  constraint midpoint L28 L244.start
  constraint midpoint L25 L244.end
  constraint perpendicular L25 L244
  constraint midpoint L19 L245.start
  constraint midpoint L14 L245.end
  constraint perpendicular L14 L245
  constraint perpendicular L228 L246
  constraint midpoint L9 L247.start
  constraint midpoint L8 L247.end
  constraint perpendicular L8 L247
  constraint perpendicular L23 L248
  constraint midpoint L42 L249.start
  constraint midpoint L46 L249.end
  constraint perpendicular L29 L250
  constraint perpendicular L220 L251
  constraint midpoint L41 L252.start
  constraint midpoint L38 L252.end
  constraint perpendicular L34 L253
  constraint midpoint L48 L254.start
  constraint midpoint L47 L254.end
  constraint perpendicular L47 L254
  constraint midpoint L240 P74
  constraint perpendicular L75 L255
  constraint midpoint L252 L256.start
  constraint perpendicular L252 L256
  constraint midpoint L253 P71
  constraint horizontal L258
  constraint perpendicular L258 L259
  constraint parallel L258 L260
  constraint parallel L259 L261
  constraint coincident L262 P63
  constraint coincident L263 P63
  constraint midpoint L229 P63
  constraint horizontal L264
  constraint perpendicular L264 L265
  constraint parallel L264 L266
  constraint parallel L265 L267
  constraint coincident L268 P64
  constraint coincident L269 P64
  constraint midpoint L231 P64
  constraint horizontal L270
  constraint perpendicular L270 L271
  constraint parallel L270 L272
  constraint parallel L271 L273
  constraint coincident L274 P65
  constraint coincident L275 P65
  constraint midpoint L234 P65
  constraint horizontal L276
  constraint perpendicular L276 L277
  constraint parallel L276 L278
  constraint parallel L277 L279
  constraint coincident L280 P66
  constraint coincident L281 P66
  constraint midpoint L236 P66
  constraint horizontal L282
  constraint perpendicular L282 L283
  constraint parallel L282 L284
  constraint parallel L283 L285
  constraint coincident L286 P67
  constraint coincident L287 P67
  constraint midpoint L246 P67
  constraint horizontal L288
  constraint perpendicular L288 L289
  constraint parallel L288 L290
  constraint parallel L289 L291
  constraint coincident L292 P68
  constraint coincident L293 P68
  constraint midpoint L247 P68
  constraint horizontal L294
  constraint perpendicular L294 L295
  constraint parallel L294 L296
  constraint parallel L295 L297
  constraint coincident L298 P69
  constraint coincident L299 P69
  constraint midpoint L250 P69
  constraint midpoint L31 L300.start
  constraint midpoint L40 L300.end
  constraint perpendicular L36 L301
  constraint horizontal L302
  constraint perpendicular L302 L303
  constraint parallel L302 L304
  constraint parallel L303 L305
  constraint coincident L306 P70
  constraint coincident L307 P70
  constraint midpoint L300 P70
  constraint horizontal L308
  constraint perpendicular L308 L309
  constraint parallel L308 L310
  constraint parallel L309 L311
  constraint coincident L312 P71
  constraint coincident L313 P71
  constraint coincident P71 L257.start
  constraint horizontal L314
  constraint perpendicular L314 L315
  constraint parallel L314 L316
  constraint parallel L315 L317
  constraint coincident L318 P72
  constraint coincident L319 P72
  constraint coincident L256 P72
  constraint coincident L251 P72
  constraint horizontal L320
  constraint perpendicular L320 L321
  constraint parallel L320 L322
  constraint parallel L321 L323
  constraint coincident L324 P73
  constraint coincident L325 P73
  constraint midpoint L242 P73
  constraint horizontal L326
  constraint perpendicular L326 L327
  constraint parallel L326 L328
  constraint parallel L327 L329
  constraint coincident L330 P74
  constraint coincident L331 P74
  constraint coincident P74 L255.start
  constraint horizontal L332
  constraint perpendicular L332 L333
  constraint parallel L332 L334
  constraint parallel L333 L335
  constraint coincident L336 P75
  constraint coincident L337 P75
  constraint midpoint L244 P75
  constraint horizontal L338
  constraint perpendicular L338 L339
  constraint parallel L338 L340
  constraint parallel L339 L341
  constraint coincident L342 P76
  constraint coincident L343 P76
  constraint midpoint L238 P76
  constraint horizontal L344
  constraint vertical L345
  constraint horizontal L346
  constraint vertical L347
  constraint coincident L62.end L72
  constraint coincident L346 L72.end
  constraint coincident L346 L348.end
  constraint perpendicular L346 L348
  constraint coincident L346 L349.end
  constraint perpendicular L346 L349
  constraint coincident L346 L350.end
  constraint perpendicular L346 L350
  constraint perpendicular L352 L353
  constraint parallel L304 L352
  constraint parallel L259 L351
  constraint coincident L55 L351.end
  constraint coincident L66 L352.start
  measures "d8" distance of L56.start L56.end
  measures "d9" distance of L56.start L58.end
  measures "d11" distance of L60.start L62.end
  measures "d12" distance of L62.end L63.end
  measures "d13" distance of L62.end L65.end
  measures "d15" distance of L62.end L69.end
  measures "d16" distance of L65.end L64.end
  measures "d17" distance of L65.end L75.end
  measures "d18" distance of L64.end L77.end
  measures "d19" distance of L64.end L63.end
  measures "d22" distance of L87.end L86.end
  measures "d23" distance of L89.start L87.end
  measures "d24" distance of L86.end L87.end
  measures "d26" distance of L97.end L96.end
  measures "d30" distance of L106.end L105.end
  measures "d34" distance of L116.end L115.end
  measures "d38" distance of L125.end L124.end
  measures "d42" distance of L135.end L134.end
  measures "d46" distance of L145.end L144.end
  measures "d47" distance of L144.end L145.start
  measures "d50" distance of L155.end L154.end
  measures "d54" distance of L165.end L164.end
  measures "d58" distance of L175.end L174.end
  measures "d62" distance of L184.end L183.end
  measures "d68" distance of L199.end L198.end
  measures "d72" distance of L209.end L208.end
  measures "d78" distance of L223.end L222.end
  measures "d97" distance of L259.end L260.end
  measures "d98" distance of L258.end L259.end
  measures "d99" distance of L265.end L266.end
  measures "d100" distance of L264.end L265.end
  measures "d101" distance of L271.end L272.end
  measures "d102" distance of L270.end L271.end
  measures "d103" distance of L277.end L278.end
  measures "d104" distance of L270.end L277.end
  measures "d105" distance of L264.start L264.end
  measures "d106" distance of L282.end L264.start
  measures "d107" distance of L258.end L258.start
  measures "d108" distance of L288.end L258.end
  measures "d109" distance of L295.end L282.start
  measures "d110" distance of L294.end L295.end
  measures "d111" distance of L303.end L288.end
  measures "d112" distance of L302.end L303.end
  measures "d113" distance of L309.end L294.end
  measures "d114" distance of L308.end L309.end
  measures "d115" distance of L315.end L316.end
  measures "d116" distance of L314.end L315.end
  measures "d117" distance of L321.end L322.end
  measures "d118" distance of L320.end L321.end
  measures "d119" distance of L322.end L328.end
  measures "d120" distance of L320.start L322.end
  measures "d121" distance of L333.end L277.end
  measures "d122" distance of L332.end L333.end
  measures "d123" distance of L277.end L278.end
  measures "d124" distance of L332.start L277.end
  measures "d127" distance of L56.start L56.end
  measures "d128" distance of L56.start L346.end
  measures "d144" distance of L65 L320
  measures "d145" distance of L58 L65
  measures "d152" distance of L64 L273
  measures "d153" distance of L57 L80
extrude "押し出し1" add sketch "スケッチ1" against normal blind 13.6 contours A0 L2 L5 L231 L232 | L2 L96 L98 L100 | L5 L6 A22 L231 L232 | A1 L2 L4 L231 L232 | L4 L6 A10 L231 L232 | L6 L101 L103 L104 | L0 A3 L11 L229 L230 | L0 L88 L89 L90 L91 L93 L95 | L0 L1 A4 L229 L230 | L3 A5 L11 L229 L230 | L1 L3 A2 L229 L230 | L3 L81 L82 L83 | A6 L7 L17 L233 L234 | L17 L110 L112 L114 | L7 A11 L15 L233 L234 | A9 L13 L17 L233 L234 | L13 L15 A19 L233 L234 | L15 L105 L107 L109 | L8 L22 A21 L247 L248 | L8 A12 L23 L247 L248 | L9 A8 L22 L247 L248 | L9 A20 L23 L247 L248 | L22 L115 L117 L119 | L23 L120 L121 L123 | L10 L14 A16 L245 L246 | L10 L124 L126 L128 | L10 A7 L19 L245 L246 | L14 A23 L228 L245 L246 | L19 A17 L228 L245 L246 | L129 L131 L133 L228 | L12 L18 A13 L235 L236 | L12 L134 L136 L138 | L12 L20 A14 L235 L236 | L16 L18 A15 L235 L236 | L16 L20 A18 L235 L236 | L16 L139 L141 L143 | L21 L31 A30 L300 L301 | L21 L144 L146 L148 | L21 A31 L40 L300 L301 | A28 L31 L36 L300 L301 | L36 L40 A47 L300 L301 | L36 L149 L151 L153 | L24 L50 A53 L241 L242 | L24 L203 L205 L207 | L24 L45 A51 L241 L242 | L44 A44 L50 L241 L242 | L44 L45 A49 L241 L242 | L44 L198 L200 L202 | L25 L37 A41 L243 L244 | L25 A37 L43 L243 L244 | L28 A38 L43 L243 L244 | L28 L37 A40 L243 L244 | L37 L164 L166 L168 | L43 L169 L171 L173 | L26 L35 A42 L227 L237 L238 | L26 L174 L175 L177 | L26 L27 A48 L227 L237 L238 | L30 L35 A36 L237 L238 | L27 L30 A35 L237 L238 | L30 L178 L180 L182 | A24 L51 L53 L239 L240 L255 | L51 L213 L214 L216 | L52 L53 A55 L239 L240 | L51 A54 L54 L239 L240 L255 | L52 A52 L54 L239 L240 | L52 L208 L210 L212 | A25 L32 L48 L253 L254 | L34 A46 L48 L253 L254 L257 | L32 L183 L185 L187 | L32 A45 L47 L253 L254 | L34 A32 L47 L253 L254 L257 | L34 L188 L190 L192 | A26 L39 L41 L251 L252 L256 | L39 L193 L195 L197 L217 L218 L220 | L41 A43 L49 L251 L252 | L38 L39 A50 L251 L252 L256 | L38 A39 L49 L251 L252 | L49 L222 L223 L224 | A27 L33 L46 L249 L250 | L33 L154 L156 L158 | L29 A29 L46 L249 L250 | L33 A33 L42 L249 L250 | L29 A34 L42 L249 L250 | L29 L159 L161 L163 | L55 L56 L62 L63 L69 L72 L344 L346 L348 | L55 L56 L62 L63 L66 L69 L70 L72 L344 L352 | L55 L56 L61 L62 L63 L67 L68 L344 L346 L348 L349 | L55 L56 L62 L63 L67 L68 L70 L344 L351 L352 L353 | L56 L58 L59 L60 L65 L66 L71 L72 L73 L76 L344 | L56 L72 L344 L346 L347 | L55 L56 L60 L61 L62 L63 L67 L70 L75 L259 L260 L289 L295 L302 L303 L304 L308 L309 L310 L314 L315 L321 L344 L351 L352 L353 | L66 L70 L72 L75 L352 | L60 L65 L70 L73 L75 L321 | L65 L66 L70 L71 L72 L73 L75 L76 | L55 L56 L63 L79 L344 L346 L349 L350 | L60 L75 L320 L321 L323 L327 | L60 L75 L317 L321 L322 L323 L327 | L56 L344 L345 L346 L350 | L55 L56 L60 L63 L75 L78 L261 L266 L267 L272 L273 L279 L317 L322 L328 L329 L332 L338 L341 L344 | L55 L56 L63 L64 L75 L78 L79 L80 L344 | L56 L57 L58 L60 L64 L65 L73 L74 L77 L80 L344 | L60 L65 L73 L75 L78 L320 L326 L329 | L60 L311 L314 L315 L316 L317 L321 | L75 L323 L327 L328 L329 | L75 L323 L326 L327 L329 | L64 L65 L73 L74 L75 L77 L78 L80 | L60 L258 L259 L260 L261 L265 L290 | L60 L294 L311 L316 L333 | L308 L309 L310 L311 L315 | L60 L261 L264 L265 L266 L267 L271 L284 L291 | L60 L297 L332 L333 L334 L335 L339 | L60 L258 L265 L285 L288 L289 L290 L291 | L60 L294 L295 L296 L297 L305 L333 | L278 L335 L338 L339 L340 L341 | L60 L264 L271 L277 L282 L283 L284 L285 L291 | L267 L270 L271 L272 L273 L276 L283 | L295 L302 L303 L304 L305 | L60 L285 L288 L296 L305 | L60 L277 L282 L297 L334 | L270 L276 L277 L278 L279 L283 L340
extrude "押し出し2" cut sketch "スケッチ1" against normal blind 11.7 contours A0 L2 L5 L231 L232 | L2 L96 L98 L100 | L5 L6 A22 L231 L232 | A1 L2 L4 L231 L232 | L4 L6 A10 L231 L232 | L6 L101 L103 L104 | L0 A3 L11 L229 L230 | L0 L88 L89 L90 L91 L93 L95 | L0 L1 A4 L229 L230 | L3 A5 L11 L229 L230 | L1 L3 A2 L229 L230 | L3 L81 L82 L83 | A6 L7 L17 L233 L234 | L17 L110 L112 L114 | L7 A11 L15 L233 L234 | A9 L13 L17 L233 L234 | L13 L15 A19 L233 L234 | L15 L105 L107 L109 | L8 L22 A21 L247 L248 | L8 A12 L23 L247 L248 | L9 A8 L22 L247 L248 | L9 A20 L23 L247 L248 | L22 L115 L117 L119 | L23 L120 L121 L123 | L10 L14 A16 L245 L246 | L10 L124 L126 L128 | L10 A7 L19 L245 L246 | L14 A23 L228 L245 L246 | L19 A17 L228 L245 L246 | L129 L131 L133 L228 | L12 L18 A13 L235 L236 | L12 L134 L136 L138 | L12 L20 A14 L235 L236 | L16 L18 A15 L235 L236 | L16 L20 A18 L235 L236 | L16 L139 L141 L143 | L21 L31 A30 L300 L301 | L21 L144 L146 L148 | L21 A31 L40 L300 L301 | A28 L31 L36 L300 L301 | L36 L40 A47 L300 L301 | L36 L149 L151 L153 | L24 L50 A53 L241 L242 | L24 L203 L205 L207 | L24 L45 A51 L241 L242 | L44 A44 L50 L241 L242 | L44 L45 A49 L241 L242 | L44 L198 L200 L202 | L25 L37 A41 L243 L244 | L25 A37 L43 L243 L244 | L28 A38 L43 L243 L244 | L28 L37 A40 L243 L244 | L37 L164 L166 L168 | L43 L169 L171 L173 | L26 L35 A42 L227 L237 L238 | L26 L174 L175 L177 | L26 L27 A48 L227 L237 L238 | L30 L35 A36 L237 L238 | L27 L30 A35 L237 L238 | L30 L178 L180 L182 | A24 L51 L53 L239 L240 L255 | L51 L213 L214 L216 | L52 L53 A55 L239 L240 | L51 A54 L54 L239 L240 L255 | L52 A52 L54 L239 L240 | L52 L208 L210 L212 | A25 L32 L48 L253 L254 | L34 A46 L48 L253 L254 L257 | L32 L183 L185 L187 | L32 A45 L47 L253 L254 | L34 A32 L47 L253 L254 L257 | L34 L188 L190 L192 | A26 L39 L41 L251 L252 L256 | L39 L193 L195 L197 L217 L218 L220 | L41 A43 L49 L251 L252 | L38 L39 A50 L251 L252 L256 | L38 A39 L49 L251 L252 | L49 L222 L223 L224 | A27 L33 L46 L249 L250 | L33 L154 L156 L158 | L29 A29 L46 L249 L250 | L33 A33 L42 L249 L250 | L29 A34 L42 L249 L250 | L29 L159 L161 L163 | L55 L56 L62 L63 L69 L72 L344 L346 L348 | L55 L56 L62 L63 L66 L69 L70 L72 L344 L352 | L55 L56 L61 L62 L63 L67 L68 L344 L346 L348 L349 | L55 L56 L62 L63 L67 L68 L70 L344 L351 L352 L353 | L55 L56 L60 L61 L62 L63 L67 L70 L75 L259 L260 L289 L295 L302 L303 L304 L308 L309 L310 L314 L315 L321 L344 L351 L352 L353 | L66 L70 L72 L75 L352 | L60 L65 L70 L73 L75 L321 | L65 L66 L70 L71 L72 L73 L75 L76 | L55 L56 L63 L79 L344 L346 L349 L350 | L60 L75 L320 L321 L323 L327 | L60 L75 L317 L321 L322 L323 L327 | L55 L56 L60 L63 L75 L78 L261 L266 L267 L272 L273 L279 L317 L322 L328 L329 L332 L338 L341 L344 | L55 L56 L63 L64 L75 L78 L79 L80 L344 | L60 L65 L73 L75 L78 L320 L326 L329 | L60 L311 L314 L315 L316 L317 L321 | L75 L323 L327 L328 L329 | L75 L323 L326 L327 L329 | L64 L65 L73 L74 L75 L77 L78 L80 | L60 L258 L259 L260 L261 L265 L290 | L60 L294 L311 L316 L333 | L308 L309 L310 L311 L315 | L60 L261 L264 L265 L266 L267 L271 L284 L291 | L60 L297 L332 L333 L334 L335 L339 | L60 L258 L265 L285 L288 L289 L290 L291 | L60 L294 L295 L296 L297 L305 L333 | L278 L335 L338 L339 L340 L341 | L60 L264 L271 L277 L282 L283 L284 L285 L291 | L267 L270 L271 L272 L273 L276 L283 | L295 L302 L303 L304 L305 | L60 L285 L288 L296 L305 | L60 L277 L282 L297 L334 | L270 L276 L277 L278 L279 L283 L340
extrude "押し出し3" add sketch "スケッチ1" against normal blind 10.5 contours L55 L56 L62 L63 L69 L72 L344 L346 L348 | L55 L56 L62 L63 L66 L69 L70 L72 L344 L352 | L66 L70 L72 L75 L352 | L60 L65 L70 L73 L75 L321 | L65 L66 L70 L71 L72 L73 L75 L76 | L55 L56 L63 L79 L344 L346 L349 L350 | L60 L75 L320 L321 L323 L327 | L55 L56 L63 L64 L75 L78 L79 L80 L344 | L60 L65 L73 L75 L78 L320 L326 L329 | L75 L323 L326 L327 L329 | L64 L65 L73 L74 L75 L77 L78 L80
extrude "押し出し4" cut sketch "スケッチ1" against normal blind 8.7 contours L55 L56 L62 L63 L69 L72 L344 L346 L348 | L55 L56 L62 L63 L66 L69 L70 L72 L344 L352 | L66 L70 L72 L75 L352 | L60 L65 L70 L73 L75 L321 | L65 L66 L70 L71 L72 L73 L75 L76 | L55 L56 L63 L79 L344 L346 L349 L350 | L60 L75 L320 L321 L323 L327 | L55 L56 L63 L64 L75 L78 L79 L80 L344 | L60 L65 L73 L75 L78 L320 L326 L329 | L75 L323 L326 L327 L329 | L64 L65 L73 L74 L75 L77 L78 L80
extrude "押し出し5" add sketch "スケッチ1" against normal blind 2.9 contours L55 L56 L62 L63 L69 L72 L344 L346 L348 | L55 L56 L62 L63 L66 L69 L70 L72 L344 L352 | L55 L56 L61 L62 L63 L67 L68 L344 L346 L348 L349 | L55 L56 L62 L63 L67 L68 L70 L344 L351 L352 L353 | L55 L56 L60 L61 L62 L63 L67 L70 L75 L259 L260 L289 L295 L302 L303 L304 L308 L309 L310 L314 L315 L321 L344 L351 L352 L353 | L66 L70 L72 L75 L352 | L60 L65 L70 L73 L75 L321 | L65 L66 L70 L71 L72 L73 L75 L76 | L55 L56 L63 L79 L344 L346 L349 L350 | L60 L75 L320 L321 L323 L327 | L60 L75 L317 L321 L322 L323 L327 | L55 L56 L60 L63 L75 L78 L261 L266 L267 L272 L273 L279 L317 L322 L328 L329 L332 L338 L341 L344 | L55 L56 L63 L64 L75 L78 L79 L80 L344 | L60 L65 L73 L75 L78 L320 L326 L329 | L60 L311 L314 L315 L316 L317 L321 | L75 L323 L327 L328 L329 | L75 L323 L326 L327 L329 | L64 L65 L73 L74 L75 L77 L78 L80 | L60 L258 L259 L260 L261 L265 L290 | L60 L294 L311 L316 L333 | L308 L309 L310 L311 L315 | L60 L261 L264 L265 L266 L267 L271 L284 L291 | L60 L297 L332 L333 L334 L335 L339 | L60 L258 L265 L285 L288 L289 L290 L291 | L60 L294 L295 L296 L297 L305 L333 | L278 L335 L338 L339 L340 L341 | L60 L264 L271 L277 L282 L283 L284 L285 L291 | L267 L270 L271 L272 L273 L276 L283 | L295 L302 L303 L304 L305 | L60 L285 L288 L296 L305 | L60 L277 L282 L297 L334 | L270 L276 L277 L278 L279 L283 L340
extrude "押し出し7" add sketch "スケッチ1" against normal blind 1.59 contours L2 L96 L98 L100 | L6 L101 L103 L104 | L0 L88 L89 L90 L91 L93 L95 | L3 L81 L82 L83 | L17 L110 L112 L114 | L15 L105 L107 L109 | L22 L115 L117 L119 | L23 L120 L121 L123 | L10 L124 L126 L128 | L129 L131 L133 L228 | L12 L134 L136 L138 | L16 L139 L141 L143 | L21 L144 L146 L148 | L36 L149 L151 L153 | L24 L203 L205 L207 | L44 L198 L200 L202 | L37 L164 L166 L168 | L43 L169 L171 L173 | L26 L174 L175 L177 | L30 L178 L180 L182 | L51 L213 L214 L216 | L52 L208 L210 L212 | L32 L183 L185 L187 | L34 L188 L190 L192 | L39 L193 L195 L197 L217 L218 L220 | L49 L222 L223 L224 | L33 L154 L156 L158 | L29 L159 L161 L163